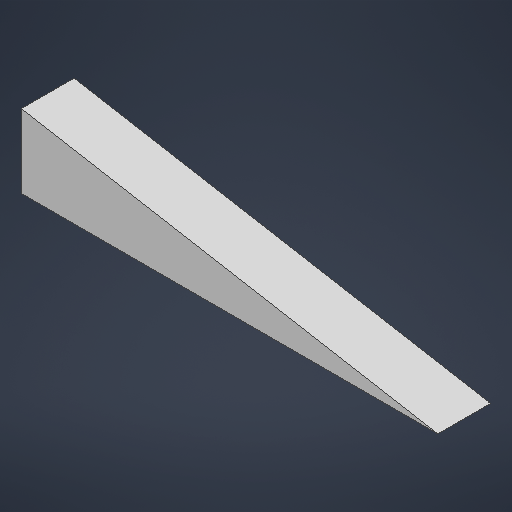
# Autodesk Inventor part: wedge
Saved by Autodesk Inventor 2026.2 (Build 302298000, 298)
## iProperties
Created: 2026-02-23
Part Number: wedge
Material: Generic
Document SubType Name: Modeling
Designer: danda
Density: 1 g/cm^3
Appearance: Default
Author: danda
Autodesk Inventor part; units mm, degrees
ref_plane "YZ Plane" through (0, 0, 0) normal (1, 0, 0) x (0, 1, 0)
ref_plane "XZ Plane" through (0, 0, 0) normal (0, 1, 0) x (-1, 0, 0)
ref_plane "XY Plane" through (0, 0, 0) normal (0, 0, 1) x (1, 0, 0)
sketch "Sketch1" plane through (0, 0, 0) normal (0, 0, 1) x (1, 0, 0)
  line L0 (12.1296, 222.6383) -> (33.4132, 218.8854)
  line L1 (12.1296, 222.6383) -> (39.6219, 222.6383) construction
  line L2 (33.4132, 218.8854) -> (12.1296, 218.8854)
  line L3 (12.1296, 218.8854) -> (12.1296, 222.6383)
  point P0 (0, 0)
  dimension "d2" = 10
  constraints: 8 end point, 2 horizontal, 1 vertical
  measures "d2" angle of L0 L1
extrude "Extrusion1" add sketch "Sketch1" along normal blind 2.7
body "Solid1"
